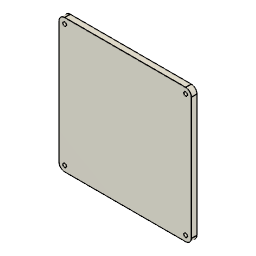
Body Door (Autodesk Fusion 360 design; units mm, degrees)
part number: 2026-07-06-14-45-42-990
Autodesk Fusion 360 part; units mm, degrees
sketch "Sketch1" plane through (0, 0, 0) normal (0, 0, 1) x (1, 0, 0)
  line L0 (0, 0) -> (115.84, 0)
  line L1 (115.84, 0) -> (115.84, 117)
  line L2 (115.84, 117) -> (0, 117)
  line L3 (0, 117) -> (0, 0)
  line L4 (10, 7) -> (105.84, 7)
  line L5 (105.84, 7) -> (105.84, 112)
  line L6 (105.84, 112) -> (10, 112)
  line L7 (10, 112) -> (10, 7)
  circle A0 centre (5, 112) radius 1.6
  circle A1 centre (5, 5) radius 1.6
  circle A2 centre (110.84, 5) radius 1.6
  circle A3 centre (110.84, 112) radius 1.6
  dimension "d1" = 115.84
  dimension "d2" = 117
  dimension "d3" = 95.84
  dimension "d4" = 105
  dimension "d6" = 10
  dimension "d7" = 5
  dimension "d8" = 3.2
  dimension "d9" = 5
  dimension "d10" = 5
  dimension "d11" = 3.2
  dimension "d12" = 5
  dimension "d13" = 5
  dimension "d14" = 3.2
  dimension "d15" = 5
  dimension "d16" = 5
  dimension "d17" = 3.2
  dimension "d18" = 5
  dimension "d19" = 5
  constraint horizontal L0
  constraint vertical L1
  constraint horizontal L2
  constraint vertical L3
  constraint coincident L0.start L3.end
  constraint horizontal L4
  constraint vertical L5
  constraint horizontal L6
  constraint vertical L7
  measures "d1" distance of L0.start L0.end
  measures "d2" distance of L0.start L2.end
  measures "d3" distance of L4.start L4.end
  measures "d4" distance of L4.start L6.end
  measures "d6" distance of L3 L7
  measures "d7" distance of L2 L6
  measures "d8" diameter of A0
  measures "d9" distance of L2 A0.centre
  measures "d10" distance of L3 A0.centre
  measures "d11" diameter of A1
  measures "d12" distance of L0 A1.centre
  measures "d13" distance of L3 A1.centre
  measures "d14" diameter of A2
  measures "d15" distance of L0 A2.centre
  measures "d16" distance of L1 A2.centre
  measures "d17" diameter of A3
  measures "d18" distance of L1 A3.centre
  measures "d19" distance of L2 A3.centre
extrude "Extrude1" add sketch "Sketch1" along normal blind 5 contours L0 L1 L2 L3 | L4 L5 L6 L7
fillet "Fillet1" radius 5 4 edges at (115.84, 117, 2.5) (115.84, 0, 2.5) (0, 117, 2.5) (0, 0, 2.5)
